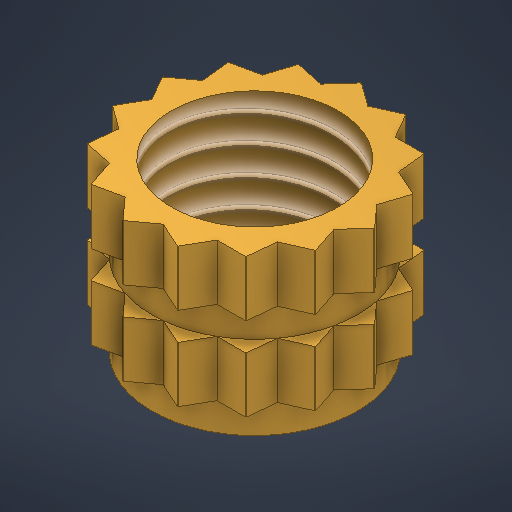
# Autodesk Inventor part: insert-M3-3x4.2
Saved by Autodesk Inventor 2026.2 (Build 302298000, 298)
## iProperties
Created: 2026-03-11
Part Number: insert-M3-3x4.2
Material: Mosiądz, miękki żółty
Document SubType Name: Modeling
Designer: idzim
Density: 8.47 g/cm^3
Appearance: Mosiądz — satynowy
Author: idzim
Autodesk Inventor part; units mm, degrees
ref_plane "YZ Plane" through (0, 0, 0) normal (1, 0, 0) x (0, 1, 0)
ref_plane "XZ Plane" through (0, 0, 0) normal (0, 1, 0) x (-1, 0, 0)
ref_plane "XY Plane" through (0, 0, 0) normal (0, 0, 1) x (1, 0, 0)
sketch "Szkic1" plane through (0, 0, 0) normal (1, 0, 0) x (0, 1, 0)
  line L0 (0, 0) -> (3, 0)
  line L1 (3, 0) -> (3, -1.5)
  line L2 (3, -1.5) -> (0, -1.5)
  line L3 (0, -1.5) -> (0, 0)
  line L4 (3, -1.5) -> (0, -1.5)
  line L5 (0, -1.5) -> (0, -1.85)
  line L6 (0, -1.85) -> (3, -1.85)
  line L7 (3, -1.85) -> (3, -1.5)
  line L8 (3, -1.5) -> (0, -1.5)
  line L9 (0, -1.5) -> (0, -2.15)
  line L10 (0, -2.15) -> (3, -2.15)
  line L11 (3, -2.15) -> (3, -1.5)
  line L12 (3, -1.85) -> (2, -1.85)
  line L13 (2, -1.85) -> (2, -2.15)
  line L14 (2, -2.15) -> (3, -2.15)
  line L15 (3, -2.15) -> (3, -1.85)
  line L16 (0.5, -2.15) -> (1.5, -2.15)
  line L17 (1.5, -2.15) -> (1.5, -1.85)
  line L18 (1.5, -1.85) -> (0.5, -1.85)
  line L19 (0.5, -1.85) -> (0.5, -2.15)
  dimension "d0" = 3
  dimension "d1" = 1.5
  dimension "d2" = 3
  dimension "d3" = 0.35
  dimension "d4" = 3
  dimension "d5" = 0.65
  dimension "d6" = 1
  dimension "d7" = 1
  dimension "d8" = 2.5
  constraints: 40 end point, 10 parallel, 5 horizontal, 5 perpendicular, 2 point on line, 1 midpoint
  measures "d0" distance of L1.end L2.end
  measures "d1" distance of L0.end L1.end
  measures "d2" distance of L6.end L5.end
  measures "d3" distance of L5.end L4.end
  measures "d4" distance of L10.end L9.end
  measures "d5" distance of L9.end L8.end
  measures "d6" distance between parallel lines of L15 L13
  measures "d7" distance between parallel lines of L19 L17
  measures "d8" distance between parallel lines of L11 L19
revolve "Obrót1" add sketch "Szkic1" angle 360 about axis through (0, 0, 0) along (0, 1, 0) contours L2 L7 L6 L5 | L11 L10 L13 L6 | L6 L17 L10 L19
thread "Gwint1" size "M3x0.5" class "6H" standard "ANSI Metric M Profile" full length
sketch "Szkic2" plane through (0, 3, 0) normal (0, 1, 0) x (1, 0, 0)
  circle A0 centre (0, 0) radius 1.85 projected
  circle A1 centre (0, 0) radius 1.5 projected
  circle A2 centre (0, 0) radius 2.15 projected
  line L0 (0, 0) -> (-2.15, 0)
  line L1 (-1.85, 0) -> (-2.1044, -0.4406)
  line L2 (-1.85, 0) -> (-2.1044, 0.4406)
  line L3 (-1.6901, -0.7525) -> (-1.7432, -1.2584)
  line L4 (-1.6901, -0.7525) -> (-2.1016, -0.4534)
  line L5 (-1.2379, -1.3748) -> (-1.0807, -1.8587)
  line L6 (-1.2379, -1.3748) -> (-1.7355, -1.269)
  line L7 (-0.5717, -1.7595) -> (-0.2313, -2.1375)
  line L8 (-0.5717, -1.7595) -> (-1.0693, -1.8652)
  line L9 (0.1934, -1.8399) -> (0.6581, -2.0468)
  line L10 (0.1934, -1.8399) -> (-0.2182, -2.1389)
  line L11 (0.925, -1.6021) -> (1.4337, -1.6021)
  line L12 (0.925, -1.6021) -> (0.6706, -2.0427)
  line L13 (1.4967, -1.0874) -> (1.9614, -0.8805)
  line L14 (1.4967, -1.0874) -> (1.4435, -1.5934)
  line L15 (1.8096, -0.3846) -> (2.15, -0.0066)
  line L16 (1.8096, -0.3846) -> (1.9668, -0.8685)
  line L17 (1.8096, 0.3846) -> (1.9668, 0.8685)
  line L18 (1.8096, 0.3846) -> (2.15, 0.0066)
  line L19 (1.4967, 1.0874) -> (1.4435, 1.5934)
  line L20 (1.4967, 1.0874) -> (1.9614, 0.8805)
  line L21 (0.925, 1.6021) -> (0.6706, 2.0427)
  line L22 (0.925, 1.6021) -> (1.4337, 1.6021)
  line L23 (0.1934, 1.8399) -> (-0.2182, 2.1389)
  line L24 (0.1934, 1.8399) -> (0.6581, 2.0468)
  line L25 (-0.5717, 1.7595) -> (-1.0693, 1.8652)
  line L26 (-0.5717, 1.7595) -> (-0.2313, 2.1375)
  line L27 (-1.2379, 1.3748) -> (-1.7355, 1.269)
  line L28 (-1.2379, 1.3748) -> (-1.0807, 1.8587)
  line L29 (-1.6901, 0.7525) -> (-2.1016, 0.4534)
  line L30 (-1.6901, 0.7525) -> (-1.7432, 1.2584)
  point P0 (-0.2182, 2.1389)
  point P1 (-0.2182, -2.1389)
  dimension "d13" = 60
  dimension "d14" = 60
  dimension "d17" = 360
  constraints: 62 end point, 1 horizontal, 1 horizontal alignment, 1 point on line, 81 other
  measures "d13" angle of L0 L1
  measures "d14" angle of L2 L0
extrude "Wyciągnięcie proste1" cut sketch "Szkic2" against normal blind 10 contours L17 A2 L18 | L15 A2 L16 | L19 A2 L20 | L13 A2 L14 | L21 A2 L22 | L11 A2 L12 | L23 A2 L24 | L9 A2 L10 | L25 A2 L26 | L7 A2 L8 | L27 A2 L28 | L5 A2 L6 | L29 A2 L30 | L3 A2 L4 | L1 A2 L0 | L0 A2 L2
